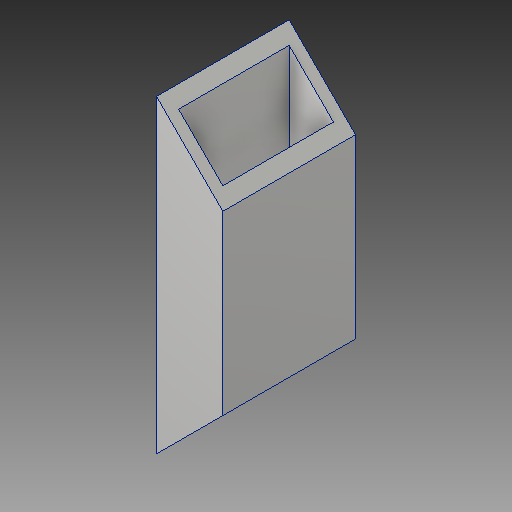
# Autodesk Inventor part: 45dege0_75x1.50ForTopOfShooter
Saved by Autodesk Inventor 2017 (Build 210142000, 142)
## iProperties
Created: 2016-02-08
Part Number: 45dege0_75x1.50ForTopOfShooter
Material: Aluminum 6061
Document SubType Name: Modeling
Designer: steele
Density: 2.7 g/cm^3
Appearance: Aluminum - Flat
Author: steele
Autodesk Inventor part; units mm, degrees
ref_plane "YZ Plane" through (0, 0, 0) normal (1, 0, 0) x (0, 1, 0)
ref_plane "XZ Plane" through (0, 0, 0) normal (0, 1, 0) x (-1, 0, 0)
ref_plane "XY Plane" through (0, 0, 0) normal (0, 0, 1) x (1, 0, 0)
sketch "Sketch1" plane through (0, 0, 0) normal (0, 0, 1) x (1, 0, 0)
  line L0 (-9.525, -25.4) -> (9.525, -25.4)
  line L1 (9.525, -25.4) -> (9.525, 25.4)
  line L2 (9.525, 25.4) -> (-9.525, 25.4)
  line L3 (-9.525, 25.4) -> (-9.525, -25.4)
  line L4 (-9.525, -25.4) -> (9.525, 25.4) construction
  line L5 (9.525, -25.4) -> (-9.525, 25.4) construction
  line L6 (9.525, 25.4) -> (-9.525, 44.45)
  line L7 (-9.525, 44.45) -> (-9.525, 25.4)
  line L8 (-9.525, -25.4) -> (-9.525, -44.45)
  line L9 (-9.525, -44.45) -> (9.525, -25.4)
  point P0 (0, 0)
  dimension "d0" = 19.05
  dimension "d1" = 45
  dimension "d2" = 45
  dimension "d10" = 88.9
  constraints: 20 end point, 2 midpoint, 2 parallel, 1 collinear, 1 horizontal, 1 perpendicular, 1 vertical
  measures "d0" distance of L0.start L0.end
  measures "d1" angle of L6 L2
  measures "d2" angle of L9 L0
  measures "d10" distance of L8.end L6.end
extrude "Extrusion1" add sketch "Sketch1" along normal mid plane 38.1
sketch "Sketch2" plane through (0, 0, 0) normal (0, 1, 0) x (-1, 0, 0)
  line L0 (6.35, 15.875) -> (-6.35, 15.875)
  line L1 (-6.35, 15.875) -> (-6.35, -15.875)
  line L2 (-6.35, -15.875) -> (6.35, -15.875)
  line L3 (6.35, -15.875) -> (6.35, 15.875)
  line L4 (6.35, 15.875) -> (-6.35, -15.875) construction
  line L5 (-6.35, 15.875) -> (6.35, -15.875) construction
  line L6 (-9.525, -19.05) -> (-9.525, 19.05) projected
  line L7 (-9.525, -19.05) -> (9.525, -19.05) projected
  point P0 (0, 0)
  dimension "d6" = 3.175
  dimension "d7" = 3.175
  constraints: 12 end point, 2 midpoint, 2 parallel, 1 horizontal, 1 perpendicular
  measures "d6" distance between parallel lines of L6 L1
  measures "d7" distance between parallel lines of L2 L7
extrude "Extrusion2" cut sketch "Sketch2" along normal through all both and the other way through all
equation "\"d0\" = width"
equation "\"d10\" = length"
equation "\"d3\" = longSide"
equation "\"d8\" = longSide"
equation "\"width\" = 19.05"
equation "\"longSide\" = 38.1"
equation "\"length\" = 88.9"
body "Solid1"
